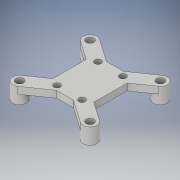
# Autodesk Inventor part: AdapterBoardNema17Mount
Saved by Autodesk Inventor 2019 (Build 230136000, 136)
## iProperties
Created: 2018-12-23
Part Number: AdapterBoardNema17Mount
Material: Generic
Document SubType Name: Modeling
Designer: Michael Wu
Density: 1 g/cm^3
Appearance: Default
Author: Michael Wu
Autodesk Inventor part; units mm, degrees
ref_plane "YZ Plane" through (0, 0, 0) normal (1, 0, 0) x (0, 1, 0)
ref_plane "XZ Plane" through (0, 0, 0) normal (0, 1, 0) x (-1, 0, 0)
ref_plane "XY Plane" through (0, 0, 0) normal (0, 0, 1) x (1, 0, 0)
sketch "Sketch1" plane through (0, 0, 0) normal (0, 1, 0) x (-1, 0, 0)
  line L0 (0, 0) -> (42.3, 0) construction
  line L1 (42.3, 0) -> (42.3, -42.3) construction
  line L2 (42.3, -42.3) -> (0, -42.3) construction
  line L3 (0, -42.3) -> (0, 0) construction
  circle A0 centre (36.65, -5.65) radius 1.7
  circle A1 centre (36.65, -36.65) radius 1.7
  circle A2 centre (5.65, -5.65) radius 1.7
  circle A3 centre (5.65, -36.65) radius 1.7
  line L4 (5.65, -5.65) -> (5.65, -36.65) construction
  line L5 (5.65, -36.65) -> (36.65, -36.65) construction
  line L6 (36.65, -36.65) -> (36.65, -5.65) construction
  line L7 (36.65, -5.65) -> (5.65, -5.65) construction
  circle A4 centre (36.65, -5.65) radius 3
  circle A5 centre (36.65, -36.65) radius 3
  circle A6 centre (5.65, -36.65) radius 3
  circle A7 centre (5.65, -5.65) radius 3
  dimension "d0" = 42.3
  dimension "d1" = 42.3
  dimension "d2" = 3.4
  dimension "d3" = 3.4
  dimension "d4" = 31
  dimension "d5" = 3.4
  dimension "d6" = 3.4
  dimension "d8" = 31
  dimension "d9" = 5.65
  dimension "d10" = 5.65
  dimension "d11" = 31
  dimension "d12" = 6
  dimension "d13" = 6
  dimension "d14" = 6
  dimension "d15" = 6
  constraints: 16 end point, 8 centre point, 4 coincident, 3 parallel, 2 perpendicular, 1 horizontal, 1 vertical
  measures "d0" distance of L1.end L2.end
  measures "d1" distance of L0.end L1.end
  measures "d2" diameter of A0
  measures "d3" diameter of A1
  measures "d4" distance of L5.end L6.end
  measures "d5" diameter of A2
  measures "d6" diameter of A3
  measures "d8" distance of L4.end L4.start
  measures "d9" distance from line of L0 L6.end
  measures "d10" distance from line of L1 L6.end
  measures "d11" distance of L5.end L4.end
  measures "d12" diameter of A4
  measures "d13" diameter of A5
  measures "d14" diameter of A6
  measures "d15" diameter of A7
extrude "Extrusion1" add sketch "Sketch1" along normal blind 4
sketch "Sketch2" plane through (-36.65, 4, -5.65) normal (0, 1, 0) x (1, 0, 0)
  line L0 (-5.65, -5.65) -> (-5.65, 36.65) construction
  line L1 (36.65, -5.65) -> (-5.65, -5.65) construction
  line L2 (-5.65, 36.65) -> (36.65, 36.65) construction
  line L3 (36.65, 36.65) -> (36.65, -5.65) construction
  line L4 (-5.65, -5.65) -> (36.65, 36.65) construction
  line L5 (-5.65, 36.65) -> (36.65, -5.65) construction
  line L6 (24.5, 4.5) -> (6.5, 4.5)
  line L7 (6.5, 4.5) -> (6.5, 26.5)
  line L8 (6.5, 26.5) -> (24.5, 26.5)
  line L9 (24.5, 26.5) -> (24.5, 4.5)
  line L10 (24.5, 4.5) -> (6.5, 26.5) construction
  line L11 (6.5, 4.5) -> (24.5, 26.5) construction
  circle A0 centre (10, 6.5) radius 1.4
  circle A1 centre (10, 24.5) radius 1.4
  circle A2 centre (21, 24.5) radius 1.4
  circle A3 centre (21, 6.5) radius 1.4
  line L12 (10, 24.5) -> (21, 24.5) construction
  line L13 (21, 24.5) -> (21, 6.5) construction
  line L14 (21, 6.5) -> (10, 6.5) construction
  line L15 (10, 6.5) -> (10, 24.5) construction
  line L16 (21, 6.5) -> (21, 4.5) construction
  line L17 (21, 24.5) -> (21, 26.5) construction
  line L18 (10, 6.5) -> (6.5, 6.5) construction
  line L19 (21, 6.5) -> (24.5, 6.5) construction
  circle A4 centre (0, 0) radius 3 projected
  circle A5 centre (0, 31) radius 3 projected
  circle A6 centre (31, 31) radius 3 projected
  circle A7 centre (31, 0) radius 3 projected
  line L20 (11.7705, 4.5) -> (1.7076, -2.4666)
  circle A8 centre (0, 0) radius 3 construction
  line L21 (6.5, 8.1488) -> (-1.7076, 2.4666)
  circle A9 centre (0, 31) radius 3 projected
  line L22 (-1.7076, 28.5334) -> (6.5, 22.8512)
  line L23 (11.7705, 26.5) -> (1.7076, 33.4666)
  line L24 (6.5, 26.5) -> (0, 31) construction
  line L25 (6.5, 4.5) -> (0, 0) construction
  line L26 (24.5, 4.5) -> (31, 0) construction
  line L27 (19.2295, 4.5) -> (29.2924, -2.4666)
  circle A10 centre (31, 0) radius 3 projected
  line L28 (32.7076, 2.4666) -> (24.5, 8.1488)
  line L29 (24.5, 26.5) -> (31, 31) construction
  line L30 (19.2295, 26.5) -> (29.2924, 33.4666)
  line L31 (24.5, 22.8512) -> (32.7076, 28.5334)
  circle A11 centre (31, 31) radius 3 projected
  arc A12 (1.7076, 33.4666) -> (-1.7076, 28.5334) centre (0, 31) ccw
  arc A13 (32.7076, 28.5334) -> (29.2924, 33.4666) centre (31, 31) ccw
  arc A14 (29.2924, -2.4666) -> (32.7076, 2.4666) centre (31, 0) ccw
  arc A15 (-1.7076, 2.4666) -> (1.7076, -2.4666) centre (0, 0) ccw
  circle A16 centre (0, 0) radius 1.7 projected
  circle A17 centre (0, 31) radius 1.7 projected
  circle A18 centre (31, 31) radius 1.7 projected
  circle A19 centre (31, 0) radius 1.7 projected
  circle A20 centre (31, 0) radius 1.7
  circle A21 centre (31, 31) radius 1.7
  circle A22 centre (0, 0) radius 1.7
  circle A23 centre (0, 31) radius 1.7
  point P0 (15.5, 15.5)
  dimension "d18" = 18
  dimension "d19" = 22
  dimension "d20" = 2.8
  dimension "d21" = 2.8
  dimension "d22" = 2.8
  dimension "d23" = 2.8
  dimension "d24" = 11
  dimension "d25" = 18
  constraints: 56 end point, 15 point on circle, 14 point on line, 12 centre point, 11 parallel, 8 coincident, 7 tangent, 6 concentric, 3 horizontal, 3 midpoint, 3 perpendicular, 2 collinear, 2 vertical, 3 other
  measures "d18" distance of L7.end L8.end
  measures "d19" distance of L6.end L7.end
  measures "d20" diameter of A0
  measures "d21" diameter of A1
  measures "d22" diameter of A2
  measures "d23" diameter of A3
  measures "d24" distance of L12.end L12.start
  measures "d25" distance of L12.start L14.end
extrude "Extrusion2" add sketch "Sketch2" along normal blind 3
body "Solid1"
